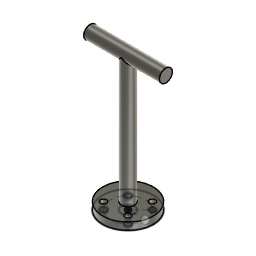
large t-handle v4 (Autodesk Fusion 360 design; units mm, degrees)
Autodesk Fusion 360 part; units mm, degrees
sketch "Sketch1" plane through (0, 0, 0) normal (0, 0, 1) x (1, 0, 0)
  circle A0 centre (0, 0) radius 35
  circle A1 centre (0, 0) radius 24 construction
  line L0 (0, 0) -> (16.9706, 16.9706) construction
  line L1 (0, 0) -> (24, 0) construction
  circle A2 centre (16.9706, 16.9706) radius 4.25
  circle A3 centre (-16.9706, 16.9706) radius 4.25
  circle A4 centre (-16.9706, -16.9706) radius 4.25
  circle A5 centre (16.9706, -16.9706) radius 4.25
  circle A6 centre (0, 0) radius 9
  dimension "d1" = 70
  dimension "d2" = 48
  dimension "d3" = 45
  dimension "d4" = 8.5
  dimension "d6" = 360
  dimension "d7" = 18
  constraint coincident A0.centre A1.centre
  constraint horizontal L1
  constraint coincident A1 L0.end
  constraint coincident L0.end A2.centre
  measures "d1" diameter of A0
  measures "d2" diameter of A1
  measures "d3" angle of L0 L1
  measures "d4" diameter of A2
  measures "d7" diameter of A6
sketch "Sketch2" plane through (0, 0, 0) normal (0, 1, 0) x (1, 0, 0)
  line L0 (-56.25, -202.5) -> (56.25, -202.5)
  line L1 (56.25, -202.5) -> (56.25, 0)
  line L2 (56.25, 0) -> (-56.25, 0)
  line L3 (-56.25, 0) -> (-56.25, -202.5)
  line L4 (0, 0) -> (0, -187.5)
  line L5 (0, -187.5) -> (52.5, -187.5)
  line L6 (0, -187.5) -> (-52.5, -187.5)
  dimension "d8" = 202.5
  dimension "d9" = 112.5
  dimension "d10" = 52.5
  dimension "d11" = 187.5
  constraint horizontal L0
  constraint vertical L1
  constraint horizontal L2
  constraint vertical L3
  constraint midpoint L2 L4.start
  constraint coincident L4.start origin
  constraint perpendicular L2 L4
  constraint perpendicular L4 L5
  constraint perpendicular L4 L6
  constraint equal L5 L6
  measures "d8" distance of L0.start L2.end
  measures "d9" distance of L0.start L0.end
  measures "d10" distance of L4.end L5.end
  measures "d11" distance of L4.start L4.end
sweep "Sweep1" add profiles "Sketch1" path "Sketch2" along L4 L5 section 1 contours A6
extrude "Extrude1" add 1 faces at (52.5, 1.9381, 188.3324) along direction (-1, 0, 0) blind 105
extrude "Extrude2" add sketch "Sketch1" along normal blind 10
equation "d8 = 135 mm * x"
equation "d9 = 75 mm * x"
equation "d10 = 35 mm * x"
equation "d11 = 125 mm * x"
equation "d18 = -70.00 mm * x"
equation "x = 1.5"
